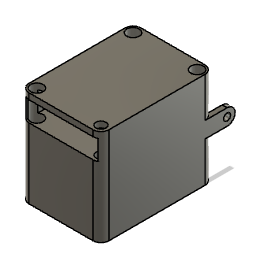
крепление камеры и аккумултора (Autodesk Fusion 360 design; units mm, degrees)
Autodesk Fusion 360 part; units mm, degrees
note: some values were not read from the file. Set by a fixed rule: which sketch regions a step uses.
sketch "Sketch1" plane through (0, 0, 0) normal (0, 1, 0) x (1, 0, 0)
  line L0 (-16, 24) -> (16, 24)
  line L1 (16, 24) -> (16, -24)
  line L2 (16, -24) -> (-16, -24)
  line L3 (-16, -24) -> (-16, 24)
  line L4 (-16, 24) -> (16, -24) construction
  line L5 (16, 24) -> (-16, -24) construction
  circle A0 centre (-16, 24) radius 2.5
  circle A1 centre (16, 24) radius 2.5
  circle A2 centre (-16, -24) radius 2.5
  circle A3 centre (16, -24) radius 2.5
  circle A4 centre (-16, -24) radius 4
  circle A5 centre (16, -24) radius 4
  circle A6 centre (16, 24) radius 4
  circle A7 centre (-16, 24) radius 4
  line L6 (-16, 24) -> (-16, 28)
  line L7 (-16, 28) -> (16, 28)
  line L8 (-16, 24) -> (-20, 24)
  line L9 (-16, -24) -> (-20, -24)
  line L10 (-20, 24) -> (-20, -24)
  line L11 (-16, -24) -> (-16, -28)
  line L12 (-16, -28) -> (16, -28)
  line L13 (16, -24) -> (20, -24)
  line L14 (20, -24) -> (20, 24)
  dimension "d1" = 32
  dimension "d2" = 48
  dimension "d3" = 5
  dimension "d4" = 5
  dimension "d5" = 5
  dimension "d6" = 5
  dimension "d7" = 8
  dimension "d8" = 8
  dimension "d9" = 8
  dimension "d10" = 8
  constraint horizontal L0
  constraint perpendicular L0 L1
  constraint parallel L0 L2
  constraint parallel L1 L3
  constraint coincident L4 origin
  constraint coincident L5 origin
  constraint coincident L0.start L3.end
  constraint coincident L0.end L1.start
  constraint coincident L2.end L3.start
  constraint coincident L1.end L2.start
  constraint concentric A2 A4
  constraint concentric A3 A5
  constraint concentric A1 A6
  constraint concentric A0 A7
  constraint coincident A7 L6.end
  constraint vertical L6
  constraint coincident A6 L7.end
  constraint tangent A6 L7
  constraint coincident A7 L8.end
  constraint parallel L7 L8
  constraint coincident A4 L9.end
  constraint perpendicular L3 L9
  constraint coincident A4 L11.end
  constraint parallel L10 L11
  constraint coincident A5 L12.end
  constraint tangent A5 L12
  constraint coincident A5 L13.end
  constraint parallel L12 L13
  constraint coincident A6 L14.end
  constraint tangent A6 L14
  measures "d1" distance of L1.end L2.end
  measures "d2" distance of L0.end L1.end
  measures "d3" diameter of A0
  measures "d4" diameter of A1
  measures "d5" diameter of A2
  measures "d6" diameter of A3
  measures "d7" diameter of A4
  measures "d8" diameter of A5
  measures "d9" diameter of A6
  measures "d10" diameter of A7
extrude "Extrude1" add sketch "Sketch1" along normal blind 8 contours L0 A0 A7 L6 | L0 L3 A0 A7 | L3 A0 A7 L8 | A0 A7 L6 L8 | L0 A6 A7 L7 | L0 L1 L2 L3 A4 A5 A6 A7 | L3 A4 A7 L10 | L0 L1 A1 A6 | L0 L1 A1 A6 | L2 L3 A2 A4 | L3 A2 A4 L9 | A2 A4 L9 L11 | L1 A5 A6 L14 | L2 A2 A4 L11 | L2 A4 A5 L12 | L1 A3 A5 L13 | L1 L2 A3 A5 | L2 A3 A5 L13
sketch "Sketch2" plane through (0, 0, 0) normal (0, -1, 0) x (1, 0, 0)
  circle A0 centre (16, 24) radius 2.5
  circle A1 centre (-16, 24) radius 2.5
  circle A2 centre (-16, -24) radius 2.5
  circle A3 centre (16, -24) radius 2.5
  arc A4 (-20, -24) -> (-16, -28) centre (-16, -24) ccw
  line L0 (-16, -28) -> (16, -28)
  arc A5 (16, -28) -> (20, -24) centre (16, -24) ccw
  line L1 (20, -24) -> (20, 24)
  arc A6 (20, 24) -> (16, 28) centre (16, 24) ccw
  line L2 (16, 28) -> (-16, 28)
  arc A7 (-16, 28) -> (-20, 24) centre (-16, 24) ccw
  line L3 (-20, 24) -> (-20, -24)
  circle A8 centre (-16, -24) radius 3.2
  circle A9 centre (16, -24) radius 3.2
  circle A10 centre (-16, 24) radius 3.2
  circle A11 centre (16, 24) radius 3.2
  dimension "d13" = 6.4
  dimension "d14" = 6.4
  dimension "d15" = 6.4
  dimension "d16" = 6.4
  constraint concentric A2 A8
  constraint concentric A3 A9
  constraint concentric A1 A10
  constraint concentric A0 A11
  measures "d13" diameter of A8
  measures "d14" diameter of A9
  measures "d15" diameter of A10
  measures "d16" diameter of A11
extrude "Extrude2" cut sketch "Sketch2" against normal blind 2.5 contours A8 | A9 | A10 | A11
sketch "Sketch3" plane through (0, 8, 0) normal (0, 1, 0) x (-1, 0, 0)
  circle A0 centre (-16, 24) radius 2.5
  circle A1 centre (16, 24) radius 2.5
  circle A2 centre (16, -24) radius 2.5
  circle A3 centre (-16, -24) radius 2.5
  arc A4 (16, -28) -> (20, -24) centre (16, -24) ccw
  line L0 (20, -24) -> (20, 24)
  arc A5 (20, 24) -> (16, 28) centre (16, 24) ccw
  line L1 (16, 28) -> (-16, 28)
  arc A6 (-16, 28) -> (-20, 24) centre (-16, 24) ccw
  line L2 (-20, 24) -> (-20, -24)
  arc A7 (-20, -24) -> (-16, -28) centre (-16, -24) ccw
  line L3 (-16, -28) -> (16, -28)
  circle A8 centre (16, -24) radius 3.125
  circle A9 centre (-16, -24) radius 3.125
  circle A10 centre (16, 24) radius 3.125
  dimension "d19" = 6.25
  dimension "d20" = 6.25
  dimension "d21" = 6.25
  constraint concentric A2 A8
  constraint concentric A3 A9
  constraint concentric A1 A10
  measures "d19" diameter of A8
  measures "d20" diameter of A9
  measures "d21" diameter of A10
extrude "Extrude3" add sketch "Sketch3" along normal blind 35 contours A4 L0 A5 L1 A6 L2 A7 L3
extrude "Extrude4" add 1 faces at (5.0453, 43, 7.366) along direction (0, 1, 0) blind 5
sketch "Sketch4" plane through (0, 0, 28) normal (0, 0, 1) x (1, 0, 0)
  line L0 (-16, 0) -> (16, 0)
  line L1 (16, 0) -> (16, 48)
  line L2 (16, 48) -> (-16, 48)
  line L3 (-16, 48) -> (-16, 0)
  line L4 (-18, 45) -> (18, 45)
  line L5 (18, 45) -> (18, 35)
  line L6 (18, 35) -> (-18, 35)
  line L7 (-18, 35) -> (-18, 45)
  line L8 (-18, 45) -> (18, 35) construction
  line L9 (18, 45) -> (-18, 35) construction
  point P0 (0, 40)
  constraint horizontal L4
  constraint perpendicular L4 L5
  constraint parallel L4 L6
  constraint parallel L5 L7
  constraint coincident L8 P0
  constraint coincident L9 P0
extrude "Extrude5" cut sketch "Sketch4" against normal blind 50 contours L3 L4 L6 L7 | L1 L3 L4 L6 | L1 L4 L5 L6
sketch "Sketch5" plane through (-20, 0, 0) normal (-1, 0, 0) x (0, 0, 1)
  line L0 (-24, 0) -> (24, 0)
  line L1 (24, 0) -> (24, 48)
  line L2 (24, 48) -> (-24, 48)
  line L3 (-24, 48) -> (-24, 0)
  line L4 (-24, 0) -> (-24, 24)
  line L5 (-24, 24) -> (-35, 24)
  circle A0 centre (-35, 24) radius 1.75
  circle A1 centre (-35, 24) radius 4
  line L6 (-35, 24) -> (-35, 28)
  line L7 (-35, 24) -> (-35, 20)
  line L8 (-35, 20) -> (-24, 20)
  line L9 (-35, 28) -> (-24, 28)
  dimension "d28" = 3.5
  dimension "d29" = 8
  constraint coincident L0.start L3.end
  constraint midpoint L3 L4.end
  constraint perpendicular L3 L5
  constraint coincident L5.end A0.centre
  constraint concentric A0 A1
  constraint coincident A1 L6.end
  constraint perpendicular L5 L6
  constraint coincident A1 L7.end
  constraint parallel L6 L7
  constraint coincident L4 L8.end
  constraint coincident L3 L9.end
  constraint tangent A1 L9
  measures "d28" diameter of A0
  measures "d29" diameter of A1
extrude "Extrude6" add sketch "Sketch5" against normal blind 2.5 contours L3 L4 L5 A1 L8 | L3 L5 A1 L9 | L5 A0 A1 L7 | A0 A1 L6 L7 | L5 A0 A1 L6
sketch "Sketch6" plane through (20, 0, 0) normal (1, 0, 0) x (0, 0, -1)
  line L0 (-24, 0) -> (24, 0)
  line L1 (24, 0) -> (24, 48)
  line L2 (24, 48) -> (-24, 48)
  line L3 (-24, 48) -> (-24, 0)
  line L4 (24, 24) -> (35, 24)
  circle A0 centre (35, 24) radius 1.75
  circle A1 centre (35, 24) radius 4
  line L5 (35, 24) -> (35, 28)
  line L6 (35, 24) -> (35, 20)
  line L7 (35, 20) -> (24, 20)
  line L8 (35, 28) -> (24, 28)
  dimension "d32" = 3.5
  constraint midpoint L1 L4.start
  constraint perpendicular L1 L4
  constraint coincident L4.end A0.centre
  constraint concentric A0 A1
  constraint coincident A1 L5.end
  constraint perpendicular L4 L5
  constraint coincident A1 L6.end
  constraint parallel L5 L6
  constraint coincident L1 L7.end
  constraint perpendicular L1 L7
  constraint coincident L1 L8.end
  constraint tangent A1 L8
  constraint perpendicular L1 L8
  measures "d32" diameter of A0
extrude "Extrude7" add sketch "Sketch6" against normal blind 2.5 contours L1 L4 A1 L7 | L1 L4 A1 L8 | A0 A1 L5 L6 | L4 A0 A1 L6 | L4 A0 A1 L5
sketch "Sketch7" plane through (0, 0, 0) normal (0, -1, 0) x (1, 0, 0)
  circle A0 centre (16, 24) radius 3.2
  circle A1 centre (-16, -24) radius 3.2
  circle A2 centre (-16, 24) radius 3.2
  circle A3 centre (16, -24) radius 3.2
  arc A4 (-20, -24) -> (-16, -28) centre (-16, -24) ccw
  line L0 (-16, -28) -> (16, -28)
  arc A5 (16, -28) -> (20, -24) centre (16, -24) ccw
  line L1 (20, -24) -> (20, 24)
  arc A6 (20, 24) -> (16, 28) centre (16, 24) ccw
  line L2 (16, 28) -> (-16, 28)
  arc A7 (-16, 28) -> (-20, 24) centre (-16, 24) ccw
  line L3 (-20, 24) -> (-20, -24)
  line L4 (16, -18) -> (-16, -18)
  line L5 (-16, -18) -> (-16, 18)
  line L6 (-16, 18) -> (16, 18)
  line L7 (16, 18) -> (16, -18)
  line L8 (16, -18) -> (-16, 18) construction
  line L9 (-16, -18) -> (16, 18) construction
  constraint horizontal L4
  constraint perpendicular L4 L5
  constraint parallel L4 L6
  constraint parallel L5 L7
  constraint coincident L8 origin
  constraint coincident L9 origin
extrude "Extrude8" cut sketch "Sketch7" against normal blind 24 contours L4 L5 L6 L7
